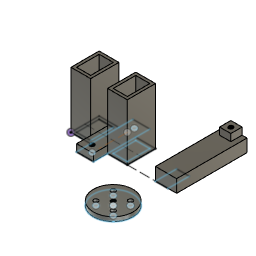
Brush_holder v1 (Autodesk Fusion 360 design; units mm, degrees)
Autodesk Fusion 360 part; units mm, degrees
sketch "Sketch1" plane through (0, 0, 0) normal (0, 0, 1) x (1, 0, 0)
  line L0 (40, 0) -> (40, 20)
  line L1 (0, 20) -> (0, 0)
  line L2 (20, 20) -> (20, 0) construction
  line L3 (0, 10) -> (40, 10) construction
  line L4 (26, 0) -> (26, -10)
  line L5 (26, -10) -> (14, -10)
  line L6 (14, -10) -> (14, 0)
  line L7 (14, 30) -> (14, 20)
  line L8 (26, 30) -> (14, 30)
  line L9 (26, 20) -> (26, 30)
  line L10 (0, 0) -> (14, 0)
  line L11 (26, 0) -> (40, 0)
  line L12 (40, 20) -> (26, 20)
  line L13 (14, 20) -> (0, 20)
  line L14 (12, 18) -> (2, 18)
  line L15 (2, 18) -> (2, 2)
  line L16 (2, 2) -> (12, 2)
  line L17 (28, 18) -> (38, 18)
  line L18 (38, 18) -> (38, 2)
  line L19 (38, 2) -> (28, 2)
  line L20 (2, 18) -> (12, 18)
  line L21 (12, 2) -> (12, 18)
  line L22 (28, 2) -> (28, 18)
  circle A0 centre (20, -5) radius 1.5
  circle A1 centre (20, 25) radius 1.5
  line L23 (14, 20) -> (14, 0)
  line L24 (26, 20) -> (26, 0)
  line L25 (40, 0) -> (60, 0) construction
  line L26 (60, 0) -> (69, 0)
  line L27 (69, 0) -> (69, 15)
  line L28 (69, 15) -> (60, 15)
  line L29 (60, 15) -> (60, 0)
  circle A2 centre (60, -30) radius 14
  circle A3 centre (60, -30) radius 1.5
  circle A4 centre (53.85, -23.85) radius 1.6
  circle A5 centre (66.15, -23.85) radius 1.6
  circle A6 centre (53.85, -36.15) radius 1.6
  circle A7 centre (66.15, -36.15) radius 1.6
  dimension "d1" = 40
  dimension "d2" = 20
  dimension "d3" = 10
  dimension "d5" = 3
  dimension "d10" = 9
  dimension "d11" = 15
  dimension "d21" = 28
  dimension "d25" = 12.3
  dimension "d26" = 3
  dimension "d27" = 3.2
  dimension "d28" = 3.2
  dimension "d29" = 3.2
  dimension "d30" = 3.2
  constraint horizontal L10
  constraint vertical L0
  constraint horizontal L12
  constraint vertical L1
  constraint coincident L1.end L10.start
  constraint midpoint L1 L3.start
  constraint midpoint L0 L3.end
  constraint coincident L4.start L10
  constraint perpendicular L4 L10
  constraint perpendicular L4 L5
  constraint perpendicular L6 L10
  constraint symmetric L3 L6.end L7.end
  constraint symmetric L3 L4.start L9.start
  constraint symmetric L3 L4.end L8.start
  constraint symmetric L3 L5.end L7.start
  constraint collinear L10 L11
  constraint coincident L2.end L10
  constraint collinear L12 L13
  constraint symmetric L2 L14.end L17.end
  constraint symmetric L2 L15.end L18.end
  constraint perpendicular L15 L20
  constraint perpendicular L20 L21
  constraint symmetric L2 L14.start L17.start
  constraint symmetric L2 L16.end L19.end
  constraint symmetric L3 A0 A1
  constraint perpendicular L0 L25
  constraint horizontal L26
  constraint vertical L27
  constraint horizontal L28
  constraint vertical L29
  constraint concentric A2 A3
  measures "d1" distance of L1.end L0.start
  measures "d2" distance of L0.start L0.end
  measures "d3" distance of L4.start L4.end
  measures "d5" diameter of A0
  measures "d10" distance of L25.end L26.end
  measures "d11" distance of L26.end L27.end
  measures "d21" diameter of A2
  measures "d25" distance of A4.centre A6.centre
  measures "d26" diameter of A3
  measures "d27" diameter of A4
  measures "d28" diameter of A5
  measures "d29" diameter of A6
  measures "d30" diameter of A7
extrude "Extrude1" add sketch "Sketch1" along normal blind 2 contours L4 L5 L6 L7 L8 L9 L23 L24 makes body 1
extrude "Extrude2" add sketch "Sketch1" along normal blind 40 contours L0 L11 L12 L24 | L1 L10 L13 L23 bodies 1
extrude "Extrude3" add sketch "Sketch1" along normal blind 50 separate body contours L26 L27 L28 L29 makes body 2
sketch "Sketch2" plane through (69, 0, 0) normal (1, 0, 0) x (0, 1, 0)
  line L0 (0, 0) -> (15, 0)
  line L1 (15, 0) -> (15, 50)
  line L2 (15, 50) -> (0, 50)
  line L3 (0, 50) -> (0, 0)
  line L4 (3.5, 50) -> (11.5, 50)
  line L5 (11.5, 42) -> (3.5, 42)
  line L6 (3.5, 45) -> (15, 45) construction
  line L7 (7.5, 50) -> (7.5, 42) construction
  circle A0 centre (7.5, 46) radius 1.5
  line L8 (7.5, 50) -> (3.5, 50)
  line L9 (3.5, 50) -> (3.5, 42)
  line L10 (11.5, 50) -> (11.5, 42)
  line L11 (7.5, 50) -> (7.5, 46)
  dimension "d17" = 3
  dimension "d18" = 4
  dimension "d39" = 8
  constraint horizontal L4
  constraint horizontal L5
  constraint perpendicular L6 L7
  constraint midpoint L7 A0.centre
  constraint perpendicular L7 L8
  constraint perpendicular L5 L9
  constraint symmetric L7 L4.start L4.end
  constraint symmetric L7 L5.end L5.start
  constraint coincident L4 L7.start
  constraint coincident L9 L6.start
  constraint coincident L7 A0.centre
  constraint perpendicular L4 L11
  constraint coincident A0.centre L11.end
  measures "d17" diameter of A0
  measures "d18" distance of L7.start L4.start
  measures "d39" distance of L4.end L5.start
extrude "Extrude4" add sketch "Sketch2" along normal blind 5 contours L2 L4 L5 L8 L9 L10 bodies 2
extrude "Extrude5" add sketch "Sketch1" along normal blind 3 separate body contours A2 makes body 3
move_body "Move1" bodies 2 to x (1, 0, 0) y (0, 0, -1) z (0, 1, 0) at (0, 15, 15)
move_body "Move2" bodies 2 to x (0, 0, 1) y (0, 1, 0) z (-1, 0, 0) at (60, 0, -60)
move_body "Move3" bodies 2 to x (1, 0, 0) y (0, 1, 0) z (0, 0, 1) at (15, -15, 0)
extrude "Extrude6" add 1 faces at (18, 13.3333, 2) along direction (0, 0, 1) blind 3 on bodies 1 bodies 1
thread "Thread1" "ISO Metric profile 3.0 M3x0.5 6H" major diameter 3.086 minor diameter 2.529 pitch 0.5 angle 60 modelled right hand crest width 0.1368 on face at (21.4981, -5.0748, 3.3333) crest through (21.2645, -5, 0.125) on bodies 1
thread "Thread2" "ISO Metric profile 3.0 M3x0.5 6H" major diameter 3.086 minor diameter 2.529 pitch 0.5 angle 60 modelled right hand crest width 0.1368 on face at (18.5075, 24.8506, 3.3333) crest through (21.2645, 25, 0.125) on bodies 1
extrude "Extrude7" cut 1 faces at (66.6842, 46.2169, 9) along direction (0, 0, -1) blind 13 on bodies 2 bodies 2
thread "Thread3" "ISO Metric profile 3.0 M3x0.5 6H" major diameter 3.086 minor diameter 2.529 pitch 0.5 angle 60 modelled right hand crest width 0.1368 on face at (68.8822, 45.4173, 4.6667) crest through (68.7645, 46, 0.125) on bodies 2
thread "Thread4" "ISO Metric profile 3.0 M3x0.5 6H" major diameter 3.086 minor diameter 2.529 pitch 0.5 angle 60 modelled right hand crest width 0.1368 on face at (60.4063, -28.5561, 2) crest through (61.2645, -30, 0.125) on bodies 3
